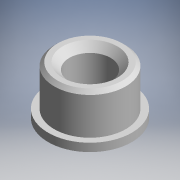
# Autodesk Inventor part: 52008.48
Saved by Autodesk Inventor 2017.3 (Build 213256000, 256)
## iProperties
Part Number: 52008.48
Material: Generic
Catalog Web Link: www.cadenas.de
Description: WB-Wheel Bearing
Vendor: COLSONGROUP
Document SubType Name: Modeling
Designer: partserver
Manufacturer: COLSONGROUP
Mass: 4.47471 g
Surface Area: 25.3346 cm^2
Volume: 4.47471 cm^3
Density: 1 g/cm^3
Appearance: PSOLRGB-239-239-239
Category: PARTsolutions
Company: COLSONGROUP
Title: 52008.48
Author: Cadenas PARTsolutions
Comments: Wheel Bearing
PSOL_IDENT_0: {$CADENAS_DATA\23d-libs\colsongroup\colson\wheels\accessories\colson_bearings.prj},153 {VTYP=3D},{NB=
PSOL_IDENT_1: 52008.48},{LINA=52008.48},{NN=WB},{DATE=10.12.2018 11:02:41},{GEOMDATE=07.04.2017 05:36:40},{VERSION=
PSOL_IDENT_2: },{LINEID=200},{WBVAR=},{WBNUMERIC=}  {NB=52008.48},{LINA=52008.48},{KT=DUMMY},{PN=52008.48},{WB=Del
PSOL_IDENT_3: rin},{LR=0.0000},{ODR=0.0000},{IDR=0.0000},{LB=0.0000},{TB=0.0000},{DB=0.0000},{ODB=0.0000},{IDB=0.0
PSOL_IDENT_4: 000},{CB=0.0000},{LD=0.6150},{TD=0.1030},{DD=1.0600},{ODD=0.9050},{IDD=0.5220},{CD=0.0600},{NOTED=1}
PSOL_IDENT_5: ,{LBB=0.00000},{TBB=0.0000},{DBB=0.0000},{ODBB=0.0000},{IDBB=0.0000},{T1BB=0.0000},{T2BB=0.0000},{CO
PSOL_IDENT_6: LOR=0.94,0.94,0.94,0.00}
NB: 52008.48
NN: WB
NT: Wheel Bearing
NBSYN: $PN.
LINA: 52008.48
CATALOG: Colson Group
PN: 52008.48
WB: Delrin
SUPPLIER: COLSONGROUP
ARTICLENO: 52008.48
BOMINFO: 52008.48
CREATOR: CADENAS GmbH
Autodesk Inventor part; units mm, degrees
sketch "Sketch_2" plane through (0, 0, 0) normal (1, 0, 0) x (0, 1, 0)
  line L0 (0, -13.0048) -> (0, 2.6162)
  line L1 (8.7847, 2.6162) -> (6.6294, 0.4609)
  line L2 (6.6294, 0.4609) -> (6.6294, -10.8495)
  line L3 (6.6294, -10.8495) -> (8.7847, -13.0048)
  line L4 (8.7847, -13.0048) -> (10.4159, -13.0048)
  line L5 (10.4159, -13.0048) -> (11.4935, -11.9272)
  line L6 (11.4935, -11.9272) -> (11.4935, 0)
  line L7 (11.4935, 0) -> (13.462, 0)
  line L8 (13.462, 0) -> (13.462, 2.6162)
  line L9 (13.462, 2.6162) -> (8.7847, 2.6162)
  constraints: 20 end point
revolve "Revolution1" add sketch "Sketch_2" angle 360 about axis through (0, 0, -13.0048) along (0, 0, -1)
ref_plane "bearings_XY" through (0, 0, 0) normal (0, 0, 1) x (1, 0, 0)
ref_plane "bearings_YZ" through (0, 0, 0) normal (1, 0, 0) x (0, 1, 0)
ref_plane "bearings_ZX" through (0, 0, 0) normal (0, 1, 0) x (0, 0, 1)
ref_plane "to_washer1_XY" through (0, 0, 0) normal (0, 0, 1) x (1, 0, 0)
ref_plane "to_washer1_YZ" through (0, 0, 0) normal (1, 0, 0) x (0, 1, 0)
ref_plane "to_washer1_ZX" through (0, 0, 0) normal (0, 1, 0) x (0, 0, 1)
ref_plane "to_washer2_XY" through (0, 0, 0) normal (0, 0, 1) x (1, 0, 0)
ref_plane "to_washer2_YZ" through (0, 0, 0) normal (1, 0, 0) x (0, 1, 0)
ref_plane "to_washer2_ZX" through (0, 0, 0) normal (0, 1, 0) x (0, 0, 1)
body "Solid1"
